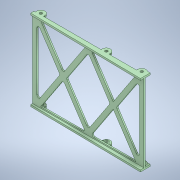
# Autodesk Inventor part: BodyStructure Plate
Saved by Autodesk Inventor 2022.2 (Build 262287030, 287C)
## iProperties
Created: 2019-11-07
Part Number: BodyStructure Plate
Material: solidworks materials|ABS
Document SubType Name: Modeling
Designer: Jochen
Density: 1.02 g/cm^3
Appearance: 151,157,178
Sending System: SolidWorks 2017
Last Author: Felix
Last Saved: 2021-02-23
Author: Jochen
Autodesk Inventor part; units mm, degrees
ref_plane "YZ Plane" through (0, 0, 0) normal (1, 0, 0) x (0, 1, 0)
ref_plane "XZ Plane" through (0, 0, 0) normal (0, 1, 0) x (-1, 0, 0)
ref_plane "Work Plane1" through (0, 0, 30) normal (0, 0, 1) x (1, 0, 0)
sketch "Sketch1" plane through (0, 0, 30) normal (0, 0, 1) x (1, 0, 0)
  line L0 (-26, -45.75) -> (26, -45.75)
  line L1 (26, 45.75) -> (-26, 45.75)
  line L2 (26, 42) -> (26, 42)
  line L3 (0, -64.05) -> (0, 64.05) construction
  line L4 (-125.2, 0) -> (51.2, 0) construction
  line L5 (-8.7414, -3.608) -> (-34.3131, -42.25)
  line L6 (-37, -37.25) -> (-12.3494, 0)
  line L7 (-37, 37.25) -> (-12.3494, 0)
  line L8 (-8.7414, 3.608) -> (-34.3131, 42.25)
  line L9 (26, -37) -> (26, -37)
  line L10 (26, -45.75) -> (26, -37)
  line L11 (26, 42) -> (26, 45.75)
  line L12 (26, -37) -> (26, 42)
  line L13 (21, -39.4907) -> (21, 39.4907)
  line L14 (21, -39.4907) -> (-5.1334, 0)
  line L15 (-5.1334, 0) -> (21, 39.4907)
  line L16 (-26, 45.75) -> (-100, 45.75)
  line L17 (-100, 45.75) -> (-100, -45.75)
  line L18 (-100, -45.75) -> (-26, -45.75)
  line L19 (-65.2586, 3.608) -> (-39.6869, 42.25)
  line L20 (-65.2586, -3.608) -> (-39.6869, -42.25)
  line L21 (-37, -37.25) -> (-61.6506, 0)
  line L22 (-37, 37.25) -> (-61.6506, 0)
  line L23 (-95, 39.4907) -> (-68.8666, 0)
  line L24 (-95, -39.4907) -> (-68.8666, 0)
  line L25 (-95, 39.4907) -> (-95, -39.4907)
  line L26 (-37, -45.75) -> (-37, 45.75) construction
  arc A0 (-39.6869, 42.25) -> (-34.3131, 42.25) centre (-37, 40.4719) ccw construction
  line L27 (-65.2586, -45.75) -> (-65.2586, 45.75) construction
  circle A1 centre (-65.2586, 0) radius 3.608 construction
  line L28 (-65.2586, 3.608) -> (-90.8303, 42.25)
  line L29 (-65.2586, -3.608) -> (-90.8303, -42.25)
  line L30 (-39.6869, 42.25) -> (-90.8303, 42.25)
  line L31 (-39.6869, -42.25) -> (-90.8303, -42.25)
  line L32 (-90.8303, 42.25) -> (-95, 42.25) construction
  line L33 (-95, 42.25) -> (-95, 39.4907) construction
  arc A2 (-95, 39.4907) -> (-90.8303, 42.25) centre (-92.9152, 40.8703) ccw construction
  line L34 (16.8303, 42.25) -> (-8.7414, 3.608)
  line L35 (-8.7414, 42.25) -> (-8.7414, -42.25) construction
  line L36 (-8.7414, -3.608) -> (16.8303, -42.25)
  line L37 (16.8303, -42.25) -> (-34.3131, -42.25)
  line L38 (-34.3131, 42.25) -> (16.8303, 42.25)
  point P0 (0, 0)
  point P1 (0, 3.7162)
  point P2 (-52.4727, 22.929)
  dimension "d7" = 91.5
  dimension "d136" = 5
  dimension "d138" = 5
  dimension "d149" = 126
  dimension "d150" = 26
  dimension "d152" = 63
  dimension "d153" = 5
  dimension "d156" = 3.5
  constraints: 75 end point, 13 point on line, 11 parallel, 8 horizontal, 8 point on circle, 7 perpendicular, 4 midpoint, 4 tangent, 3 centre point, 3 collinear, 3 vertical, 2 equal length, 8 other
  measures "d7" distance between parallel lines of L1 L0
  measures "d136" distance between parallel lines of L13 L12
  measures "d138" distance between parallel lines of L17 L25
  measures "d149" distance between parallel lines of L17 L12
  measures "d150" distance from line of L3 L1.start
  measures "d152" distance between parallel lines of L26 L12
  measures "d153" distance between parallel lines of L22 L19
  measures "d156" distance between parallel lines of L1 L38
extrude "Extrusion1" add sketch "Sketch1" along normal blind 13
fillet "Fillet1" radius 2 15 edges at (-34.3131, -42.25, 36.5) (-12.3494, 0, 36.5) (-34.3131, 42.25, 36.5) (-5.1334, 0, 36.5) (21, -39.4907, 36.5) (-37, 37.25, 36.5) (21, 39.4907, 36.5) (-65.2586, -3.608, 36.5) (-95, 39.4907, 36.5) (-61.6506, 0, 36.5) (-65.2586, 3.608, 36.5) (-68.8666, 0, 36.5) (-39.6869, -42.25, 36.5) (-95, -39.4907, 36.5) (-37, -37.25, 36.5)
sketch "Sketch3" plane through (0, 0, 0) normal (1, 0, 0) x (0, 1, 0)
  line L0 (0, -8.6) -> (0, 51.6) construction
  line L1 (-63.794, 0) -> (63.7157, 0) construction
  line L2 (-45.75, 43) -> (45.75, 43) construction
  line L3 (45.75, 43) -> (-45.75, 43) construction
  line L4 (45.75, 30) -> (-45.75, 30) construction
  line L5 (-45.75, 30) -> (45.75, 30) construction
  line L6 (45.75, 30) -> (45.75, 43) construction
  line L7 (45.75, 30) -> (45.75, 43) construction
  line L8 (37, 30) -> (37, 42.5) construction
  line L9 (37, 30) -> (37, 42.5) construction
  line L10 (-45.75, 30) -> (-45.75, 43) construction
  line L11 (-45.75, 30) -> (-45.75, 43) construction
  line L12 (-37, 30) -> (-37, 41) construction
  line L13 (-45.75, 30) -> (-45.75, 38.5)
  line L14 (-45.75, 43) -> (-45.25, 43)
  line L15 (-43.75, 39) -> (43.75, 39)
  line L16 (45.75, 40.0648) -> (45.75, 30)
  line L17 (-45.5, 43) -> (-45.5, 30) construction
  line L18 (-45.75, 43) -> (-45.75, 38.5)
  line L19 (-43.75, 30) -> (-43.75, 37.5)
  line L20 (-43.75, 37.5) -> (-42.25, 37.5)
  line L21 (40.5, 30) -> (40.5, 43) projected
  line L22 (45.75, 40.0648) -> (45.75, 43)
  line L23 (45.75, 43) -> (45, 43)
  line L24 (45.75, 43) -> (-45.75, 43) projected
  line L25 (43.75, 37.5) -> (43.75, 30)
  line L26 (31.7796, 37.5) -> (43.75, 37.5)
  line L27 (-42.25, 37.5) -> (31.7796, 37.5)
  line L28 (-45.8283, 30) -> (-43.75, 30)
  line L29 (45.75, 30) -> (-45.75, 30) projected
  line L30 (43.75, 39) -> (43.75, 43)
  line L31 (-43.75, 39) -> (-43.75, 43)
  line L32 (-45.75, 43) -> (45.75, 43) projected
  point P0 (0, 0)
  point P1 (37, 41)
  point P2 (37, 41)
  point P3 (37, 41)
  point P4 (-37, 30)
  point P5 (1.0399, 30)
  point P6 (37, 30)
  point P7 (-37, 30)
  point P8 (-45.75, 34.25)
  point P9 (-1.0399, 30)
  point P10 (21.2913, 30)
  point P11 (20.2514, 30)
  point P12 (-20.2514, 30)
  point P13 (-21.2913, 30)
  dimension "d29" = 0.5
  dimension "d85" = 2
  dimension "d88" = 7.5
  dimension "d90" = 1.5
  dimension "d160" = 87.5
  constraints: 35 end point, 4 perpendicular, 3 collinear, 2 horizontal, 2 midpoint, 2 point on line, 1 parallel, 1 vertical, 11 other
  measures "d29" distance of L3.end L14.end
  measures "d85" distance between parallel lines of L19 L10
  measures "d88" distance of L19.start L19.end
  measures "d90" distance between parallel lines of L15 L27
  measures "d160" distance between parallel lines of L31 L30
extrude "Extrusion3" cut sketch "Sketch3" along normal through all both and the other way through all contours L13 L18 L14 L24 L31 L15 L21 L26 L27 L20 L19 L28 | L21 L15 L30 L24 L23 L22 L16 L29 L25 L26 keep common part
sketch "Sketch11" plane through (0, 0, 0) normal (0, 1, 0) x (-1, 0, 0)
  line L0 (100, 43) -> (-26, 43) construction
  line L1 (6, 30) -> (26, 30)
  line L2 (-26, 30) -> (100, 30) construction
  line L3 (-26, 43) -> (-26, 39) projected
  line L4 (-26, 43) -> (-26, 30)
  line L5 (-26, 30) -> (6, 30)
  line L6 (100, 30) -> (-26, 30) projected
  line L7 (100, 37.5) -> (95, 37.5) projected
  line L8 (95, 39) -> (100, 39) projected
  line L9 (12.7477, 37.5) -> (4.7351, 37.5) projected
  line L10 (4.7351, 37.5) -> (4.7351, 39) projected
  line L11 (4.7351, 39) -> (12.7477, 39) projected
  line L12 (-21, 37.5) -> (-26, 37.5) projected
  line L13 (-26, 37.5) -> (-26, 39) projected
  line L14 (-26, 39) -> (-21, 39) projected
  line L15 (-21, 39) -> (-21, 37.5) projected
  line L16 (100, 39) -> (100, 37.5) projected
  line L17 (95, 37.5) -> (95, 39) projected
  line L18 (69.2649, 37.5) -> (61.2523, 37.5) projected
  line L19 (61.2523, 37.5) -> (61.2523, 39) projected
  line L20 (61.2523, 39) -> (69.2649, 39) projected
  line L21 (69.2649, 39) -> (69.2649, 37.5) projected
  line L22 (12.7477, 39) -> (12.7477, 37.5) projected
  line L23 (100, 30) -> (100, 43) projected
  line L24 (100, 39) -> (100, 30)
  line L25 (100, 30) -> (26, 30)
  line L26 (-26, 43) -> (100, 41)
  point P0 (0, 0)
  point P1 (-3, 43)
  point P2 (-26, 39)
  point P3 (-26, 39)
  dimension "d158" = 2
  constraints: 12 end point, 3 point on line, 2 collinear, 1 perpendicular, 1 vertical
  measures "d158" distance of L8.end L26.end
extrude "Extrusion11" cut sketch "Sketch11" along normal through all both and the other way through all contours L5 L4 L12 L15 L14 L3 L26 L23 L8 L17 L7 L6 L1 | L4 L14 L15 L12 | L7 L17 L8 L16 | L9 L10 L11 L22 | L18 L19 L20 L21 keep common part
sketch "Sketch12" plane through (0, 0, 0) normal (0, 1, 0) x (-1, 0, 0)
  circle A0 centre (-20, 35.5) radius 1.5
  circle A1 centre (-20, 35.5) radius 3
  circle A2 centre (20, 35.5) radius 1.5
  circle A3 centre (20, 35.5) radius 3
  line L0 (-26, 37.5) -> (-26, 30) construction
  line L1 (-20, 35.5) -> (20, 35.5) construction
  arc A4 (22.8284, 32) -> (24.5, 35.5) centre (20, 35.5) ccw
  arc A5 (15.5, 35.5) -> (22.8284, 32) centre (20, 35.5) ccw
  line L2 (15.5, 37) -> (-15.5, 37)
  arc A6 (-22.8284, 32) -> (-15.5, 35.5) centre (-20, 35.5) ccw
  line L3 (24.5, 35.5) -> (24.5, 36)
  arc A7 (22.8284, 32) -> (22.8284, 32) centre (19.5074, 36.1096) ccw
  line L4 (-26, 32) -> (-22.8284, 32)
  line L5 (-26, 43) -> (-26, 32)
  line L6 (-26, 43) -> (26, 43)
  line L7 (100, 39) -> (-26, 39) projected
  line L8 (-22.8284, 39) -> (22.9247, 39)
  arc A8 (-24.5, 35.5) -> (-22.8284, 32) centre (-20, 35.5) ccw
  line L9 (15.5, 35.5) -> (15.5, 37)
  line L10 (24.5, 36) -> (24.5, 37.5)
  line L11 (24.5, 37.5) -> (22.2361, 37.5)
  line L12 (-24.5, 37) -> (-24.5, 35.5)
  line L13 (-15.5, 37) -> (-15.5, 35.5)
  line L14 (100, 37.5) -> (-26, 37.5) projected
  line L15 (-22.2361, 37.5) -> (-24.5, 37.5)
  line L16 (-24.5, 37) -> (-24.5, 37.5)
  line L17 (-17.7639, 37.5) -> (-15.5, 37.5)
  line L18 (-18.6348, 37.5) -> (-1.7039, 37.5) projected
  line L19 (-15.5, 37) -> (-15.5, 36.8517)
  line L20 (-15.5, 37) -> (-15.5, 37.5)
  line L21 (15.5, 37) -> (15.5, 37.5)
  line L22 (16.9309, 37.5) -> (-16.9309, 37.5) projected
  line L23 (15.5, 37.5) -> (17.7639, 37.5)
  line L24 (8.7414, 37.5) -> (32.2592, 37.5) projected
  circle A9 centre (94, 35.5) radius 1.5
  circle A10 centre (94, 35.5) radius 3
  arc A11 (89.5, 35.5) -> (98.5, 35.5) centre (94, 35.5) ccw
  line L25 (100, 37.5) -> (100, 30) projected
  line L26 (24.5, 37) -> (89.5, 37)
  line L27 (89.5, 37) -> (89.5, 35.5)
  line L28 (93.3278, 37.5) -> (62.783, 37.5) projected
  line L29 (89.5, 37.5) -> (91.7639, 37.5)
  line L30 (100, 37.5) -> (-26, 37.5) projected
  line L31 (96.2361, 37.5) -> (98.5, 37.5)
  line L32 (98.5, 35.5) -> (98.5, 37.5)
  line L33 (100, 37.5) -> (100, 43)
  line L34 (100, 43) -> (26, 43)
  line L35 (89.5, 37) -> (89.5, 37.5)
  point P0 (0, 0)
  point P1 (-24.4142, 32)
  point P2 (22.8284, 32)
  point P3 (17.4019, 37)
  point P4 (-17.4019, 37)
  point P5 (-22.5981, 37)
  point P6 (1.7039, 37.5)
  point P7 (18.6348, 37.5)
  point P8 (59, 39)
  point P9 (24.5, 37.5)
  point P10 (-26, 37.5)
  point P11 (98.5, 37.5)
  point P12 (89.5, 37.5)
  point P13 (24.5, 37)
  dimension "d98" = 3
  dimension "d99" = 6
  dimension "d100" = 6
  dimension "d102" = 7.5
  dimension "d110" = 4.5
  dimension "d113" = 6
  dimension "d114" = 11
  dimension "d141" = 6
  dimension "d151" = 40
  constraints: 54 end point, 21 point on circle, 15 point on line, 12 centre point, 9 vertical, 8 coincident, 8 equal radius, 7 tangent, 4 horizontal, 2 collinear, 2 perpendicular, 1 midpoint, 10 other
  measures "d98" diameter of A0
  measures "d99" diameter of A1
  measures "d100" distance from line of L1.start L0
  measures "d102" vertical distance of L5.start A0.centre
  measures "d110" radius of A4
  measures "d113" distance between parallel lines of L6 L2
  measures "d114" distance between parallel lines of L6 L4
  measures "d141" distance from line of L25 A9.centre
  measures "d151" distance of A2.centre A0.centre
extrude "Extrusion12" cut sketch "Sketch12" along normal through all both and the other way through all contours A0 | A2 | A9
extrude "Extrusion13" cut sketch "Sketch12" along normal through all both and the other way through all contours A0 | A1 L14 | A1 L14 L20 L13 A6 A8 L12 L16 | L14 A1 | A1 L14 L5 L7 A7 | L16 L12 A8 L4 L5 L14 | L14 A7 L2 L20 | L5 L6 L34 L33 L7 A7 | A7 L14 L21 L2 | A7 L7 L14 L11 A3 | L21 L14 A3 L11 L10 L3 A4 A5 L9 | A7 L7 | L7 L33 L14 A10 A7 | L26 L10 L14 A7 | A7 L14 L35 L26 | L14 A3 | A3 L14 | L35 L14 A10 L32 A11 L27 | A10 L14 | L14 A10 | A2 | A9 keep common part
extrude "Extrusion14" add sketch "Sketch12" along normal blind 1 from surface at -43.75 contours A1 L14 | A1 L14 L20 L13 A6 A8 L12 L16 | L14 A1 | L21 L14 A3 L11 L10 L3 A4 A5 L9 | L14 A3 | A3 L14 | L35 L14 A10 L32 A11 L27 | A10 L14 | L14 A10
extrude "Extrusion15" add sketch "Sketch12" against normal blind 1 from surface at 43.75 contours A1 L14 | A1 L14 L20 L13 A6 A8 L12 L16 | L14 A1 | L21 L14 A3 L11 L10 L3 A4 A5 L9 | L14 A3 | A3 L14 | L35 L14 A10 L32 A11 L27 | L14 A10 picked at (94.5816, 37.3297)
chamfer "Chamfer2" distance 1 distance2 2 1 edges at (20, -42.75, 31) measured on face at (20, -43.25, 31)
chamfer "Chamfer3" distance 1 distance2 2 1 edges at (20, 42.75, 31) measured on face at (20, 43.25, 31)
chamfer "Chamfer4" distance 2 distance2 1 2 edges at (-20, 42.75, 31) (-24.5, 42.75, 36.5) measured on face at (-24, 42.75, 36.5) measured on face at (-20, 42.75, 31.5)
chamfer "Chamfer5" distance 2 distance2 1 3 edges at (-20, -42.75, 31) (-15.5, -42.75, 36.5) (-24.5, -42.75, 36.5) measured on face at (-20, -42.75, 31.5) measured on face at (-16, -42.75, 36.5) measured on face at (-24, -42.75, 36.5)
chamfer "Chamfer6" distance 2 distance2 1 3 edges at (-94, -42.75, 31) (-89.5, -42.75, 36.5) (-98.5, -42.75, 36.5) measured on face at (-90, -42.75, 36.5) measured on face at (-98, -42.75, 36.5) measured on face at (-94, -42.75, 31.5)
chamfer "Chamfer7" distance 2 distance2 1 3 edges at (-94, 42.75, 31) (-98.5, 42.75, 36.5) (-89.5, 42.75, 36.5) measured on face at (-90, 42.75, 36.5) measured on face at (-98, 42.75, 36.5) measured on face at (-94, 42.75, 31.5)
body "Solid1"
body "Solid2"
